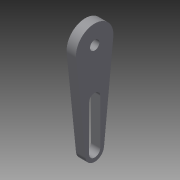
# Autodesk Inventor part: CURM_Caterpillar_leg
Saved by Autodesk Inventor 2015 (Build 190159000, 159)
## iProperties
Created: 2015-02-11
Part Number: CURM_Caterpillar_leg
Material: Generic
Document SubType Name: Modeling
Designer: Judson
Density: 1 g/cm^3
Appearance: Default
Author: Judson
Autodesk Inventor part; units mm, degrees
ref_plane "YZ Plane" through (0, 0, 0) normal (1, 0, 0) x (0, 1, 0)
ref_plane "XZ Plane" through (0, 0, 0) normal (0, 1, 0) x (-1, 0, 0)
ref_plane "XY Plane" through (0, 0, 0) normal (0, 0, 1) x (1, 0, 0)
sketch "Sketch2" plane through (0, 0, 0) normal (1, 0, 0) x (0, 1, 0)
  arc A0 (-0.648, -6.3169) -> (-0.648, 6.3169) centre (0, 0) ccw
  line L0 (6.35, 6.35) -> (-34.29, 6.35)
  line L1 (-34.29, 6.35) -> (-34.29, -6.35)
  line L2 (-34.29, -6.35) -> (6.35, -6.35)
  line L3 (6.35, -6.35) -> (6.35, 6.35)
  circle A1 centre (0, 0) radius 1.5875
  line L4 (-34.29, 0) -> (-33.02, 0)
  arc A2 (-31.115, 1.905) -> (-31.115, -1.905) centre (-31.115, 0) ccw
  arc A3 (-31.439, 3.1584) -> (-31.439, -3.1584) centre (-31.115, 0) ccw
  line L5 (-33.02, 0) -> (-13.97, 0)
  arc A4 (-15.875, -1.905) -> (-15.875, 1.905) centre (-15.875, 0) ccw
  line L6 (-15.875, -1.905) -> (-31.115, -1.905)
  line L7 (-15.875, 1.905) -> (-31.115, 1.905)
  line L8 (-0.648, -6.3169) -> (-31.439, -3.1584)
  line L9 (-0.648, 6.3169) -> (-31.439, 3.1584)
  dimension "d16" = 12.7
  dimension "d17" = 40.64
  dimension "d18" = 3.175
  dimension "d19" = 1.27
  dimension "d20" = 3.81
  dimension "d21" = 6.35
  dimension "d22" = 19.05
  dimension "d23" = 3.81
  constraints: 20 end point, 9 point on circle, 5 centre point, 5 tangent, 3 horizontal, 2 coincident, 2 parallel, 2 symmetric about line, 1 midpoint, 1 perpendicular, 1 point on line, 1 vertical
  measures "d16" diameter of A0
  measures "d17" distance of L1.end L2.end
  measures "d18" diameter of A1
  measures "d19" distance of L4.start L4.end
  measures "d20" diameter of A2
  measures "d21" diameter of A3
  measures "d22" distance of L4.end L5.end
  measures "d23" diameter of A4
extrude "Extrusion3" add sketch "Sketch2" along normal blind 3.175 contours L8 A3 L9 A0
body "Solid2"
